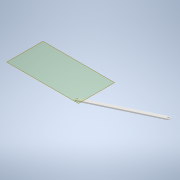
# Autodesk Inventor part: truss frame slanting down
Saved by Autodesk Inventor 2020 (Build 240168000, 168)
## iProperties
Created: 2020-07-04
Part Number: truss frame slanting down
Material: Generic
Document SubType Name: Modeling
Designer: Ashiqrahman
Density: 1 g/cm^3
Appearance: Default
Author: Ashiqrahman
Autodesk Inventor part; units mm, degrees
ref_plane "YZ Plane" through (0, 0, 0) normal (1, 0, 0) x (0, 1, 0)
ref_plane "XZ Plane" through (0, 0, 0) normal (0, 1, 0) x (-1, 0, 0)
ref_plane "XY Plane" through (0, 0, 0) normal (0, 0, 1) x (1, 0, 0)
ref_plane "Work Plane1" through (-69.7137, -17.3758, -3.1641) normal (0, -1, 0) x (1, 0, 0)
sketch "Sketch1" plane through (-69.7137, -17.3758, -3.1641) normal (0, -1, 0) x (1, 0, 0)
  arc A0 (76.7254, 32.2491) -> (73.2746, 39.4666) centre (75, 35.8579) ccw projected
  circle A1 centre (75, 35.8579) radius 2 projected
  arc A2 (223.2746, -32.2491) -> (226.7254, -39.4666) centre (225, -35.8579) ccw projected
  circle A3 centre (225, -35.8579) radius 2 projected
  line L0 (75, 35.8579) -> (225, -35.8579) construction
  line L1 (73.2746, 32.2491) -> (223.2746, -39.4666)
  line L2 (226.7254, -32.2491) -> (76.7254, 39.4666)
  arc A4 (76.7254, 39.4666) -> (73.2746, 32.2491) centre (75, 35.8579) ccw
  arc A5 (223.2746, -39.4666) -> (226.7254, -32.2491) centre (225, -35.8579) ccw
  point P0 (69.7137, 3.1641)
  point P1 (150, 0)
  point P2 (226.7254, -39.4666)
  dimension "d0" = 8
  constraints: 8 end point, 4 point on circle, 4 tangent, 2 centre point, 1 coincident, 1 concentric, 1 midpoint, 1 parallel
  measures "d0" diameter of A5
extrude "Extrusion1" add sketch "Sketch1" along normal blind 3
body "Solid1"
